Autodesk Inventor part; units mm, degrees
(part 2 of 2)
  line L250 (2.8637, 41.6829) -> (3.9176, 41.5971)
  arc A285 (2.2786, 42.8391) -> (2.0312, 43.0046) centre (2.0404, 42.7508) ccw
  line L251 (2.0312, 43.0046) -> (4.9529, 42.7667)
  arc A286 (4.9529, 42.7667) -> (4.682, 42.6434) centre (4.9028, 42.5177) ccw
  arc A287 (-0.6028, 41.7768) -> (-0.3767, 41.9297) centre (-0.6097, 42.0307) ccw
  arc A288 (-1.8939, 41.8886) -> (-1.6598, 41.7482) centre (-1.6667, 42.0021) ccw
  line L252 (-0.3767, 41.9297) -> (0.044, 42.8996)
  line L253 (-2.3665, 42.8343) -> (-1.8939, 41.8886)
  line L254 (-1.6598, 41.7482) -> (-0.6028, 41.7768)
  arc A289 (-2.3665, 42.8343) -> (-2.6303, 42.9721) centre (-2.5937, 42.7208) ccw
  line L255 (-2.6303, 42.9721) -> (0.3, 43.0515)
  arc A290 (0.3, 43.0515) -> (0.044, 42.8996) centre (0.277, 42.7985) ccw
  arc A291 (-5.1162, 41.4668) -> (-4.9079, 41.6431) centre (-5.1505, 41.7184) ccw
  arc A292 (-6.4117, 41.4383) -> (-6.1638, 41.324) centre (-6.1981, 41.5757) ccw
  line L256 (-4.9079, 41.6431) -> (-4.5945, 42.6529)
  line L257 (-6.9838, 42.3274) -> (-6.4117, 41.4383)
  line L258 (-6.1638, 41.324) -> (-5.1162, 41.4668)
  arc A293 (-6.9838, 42.3274) -> (-7.261, 42.4358) centre (-7.1974, 42.1899) ccw
  line L259 (-7.261, 42.4358) -> (-4.3565, 42.8316)
  arc A294 (-4.3565, 42.8316) -> (-4.5945, 42.6529) centre (-4.3519, 42.5776) ccw
  arc A295 (-9.5695, 40.6705) -> (-9.3815, 40.8684) centre (-9.6308, 40.917) ccw
  arc A296 (-10.8544, 40.5021) -> (-10.5956, 40.4153) centre (-10.6569, 40.6618) ccw
  line L260 (-9.3815, 40.8684) -> (-9.1792, 41.9061)
  line L261 (-11.5193, 41.3242) -> (-10.8544, 40.5021)
  line L262 (-10.5956, 40.4153) -> (-9.5695, 40.6705)
  arc A297 (-11.5193, 41.3242) -> (-11.8065, 41.402) centre (-11.7168, 41.1644) ccw
  line L263 (-11.8065, 41.402) -> (-8.9618, 42.1095)
  arc A298 (-8.9618, 42.1095) -> (-9.1792, 41.9061) centre (-8.9299, 41.8575) ccw
  arc A299 (-13.9107, 39.3975) -> (-13.7452, 39.6145) centre (-13.9983, 39.6359) ccw
  arc A300 (-15.1698, 39.0911) -> (-14.9032, 39.0328) centre (-14.9908, 39.2713) ccw
  line L264 (-13.7452, 39.6145) -> (-13.6562, 40.668)
  line L265 (-15.9197, 39.8365) -> (-15.1698, 39.0911)
  line L266 (-14.9032, 39.0328) -> (-13.9107, 39.3975)
  arc A301 (-15.9197, 39.8365) -> (-16.2137, 39.8828) centre (-16.0987, 39.6563) ccw
  line L267 (-16.2137, 39.8828) -> (-13.4621, 40.8937)
  arc A302 (-13.4621, 40.8937) -> (-13.6562, 40.668) centre (-13.4031, 40.6466) ccw
  arc A303 (-18.0888, 37.6625) -> (-17.9477, 37.8962) centre (-18.2016, 37.8901) ccw
  arc A304 (-19.3074, 37.2218) -> (-19.036, 37.1927) centre (-19.1489, 37.4203) ccw
  line L268 (-17.9477, 37.8962) -> (-17.9731, 38.9531)
  line L269 (-20.1334, 37.8817) -> (-19.3074, 37.2218)
  line L270 (-19.036, 37.1927) -> (-18.0888, 37.6625)
  arc A305 (-20.1334, 37.8817) -> (-20.4307, 37.896) centre (-20.292, 37.6833) ccw
  line L271 (-20.4307, 37.896) -> (-17.8046, 39.1985)
  arc A306 (-17.8046, 39.1985) -> (-17.9731, 38.9531) centre (-17.7192, 38.9592) ccw
  arc A307 (-22.0548, 35.486) -> (-21.9398, 35.7335) centre (-22.1916, 35.7) ccw
  arc A308 (-23.2186, 34.9161) -> (-22.9457, 34.9165) centre (-23.0825, 35.1305) ccw
  line L272 (-21.9398, 35.7335) -> (-22.0794, 36.7815)
  line L273 (-24.1111, 35.4828) -> (-23.2186, 34.9161)
  line L274 (-22.9457, 34.9165) -> (-22.0548, 35.486)
  arc A309 (-24.1111, 35.4828) -> (-24.4082, 35.4649) centre (-24.2473, 35.2684) ccw
  line L275 (-24.4082, 35.4649) -> (-21.9383, 37.0437)
  arc A310 (-21.9383, 37.0437) -> (-22.0794, 36.7815) centre (-21.8276, 36.8151) ccw
  arc A311 (-25.7622, 32.8934) -> (-25.6746, 33.152) centre (-25.9213, 33.0914) ccw
  arc A312 (-26.8576, 32.2011) -> (-26.5863, 32.231) centre (-26.7454, 32.429) ccw
  line L276 (-25.6746, 33.152) -> (-25.9267, 34.1787)
  line L277 (-27.8062, 32.668) -> (-26.8576, 32.2011)
  line L278 (-26.5863, 32.231) -> (-25.7622, 32.8934)
  arc A313 (-27.8062, 32.668) -> (-28.0996, 32.618) centre (-27.9183, 32.4401) ccw
  line L279 (-28.0996, 32.618) -> (-25.8149, 34.4545)
  arc A314 (-25.8149, 34.4545) -> (-25.9267, 34.1787) centre (-25.68, 34.2393) ccw
  point P0 (-30.4251, 30.4251)
  point P1 (-33.5363, 26.9572)
  point P2 (-36.2543, 23.1733)
  point P3 (-38.5472, 19.1177)
  point P4 (-40.3883, 14.8379)
  point P5 (-41.7558, 10.3842)
  point P6 (-42.6337, 5.8087)
  point P7 (-43.0118, 1.1652)
  point P8 (-42.8857, -3.4921)
  point P9 (-42.2567, -8.1084)
  point P10 (-41.1323, -12.6296)
  point P11 (-39.5257, -17.0027)
  point P12 (-37.4557, -21.1765)
  point P13 (-34.9465, -25.1021)
  point P14 (-32.0277, -28.7333)
  point P15 (-28.7333, -32.0277)
  point P16 (-25.1021, -34.9465)
  point P17 (-21.1765, -37.4557)
  point P18 (-17.0027, -39.5257)
  point P19 (-12.6296, -41.1323)
  point P20 (-8.1084, -42.2567)
  point P21 (-3.4921, -42.8857)
  point P22 (1.1652, -43.0118)
  point P23 (5.8087, -42.6337)
  point P24 (10.3842, -41.7558)
  point P25 (14.8379, -40.3883)
  point P26 (19.1177, -38.5472)
  point P27 (23.1733, -36.2543)
  point P28 (26.9572, -33.5363)
  point P29 (30.4251, -30.4251)
  point P30 (33.5363, -26.9572)
  point P31 (36.2543, -23.1733)
  point P32 (38.5472, -19.1177)
  point P33 (40.3883, -14.8379)
  point P34 (41.7558, -10.3842)
  point P35 (42.6337, -5.8087)
  point P36 (43.0118, -1.1652)
  point P37 (42.8857, 3.4921)
  point P38 (42.2567, 8.1084)
  point P39 (41.1323, 12.6296)
  point P40 (39.5257, 17.0027)
  point P41 (37.4557, 21.1765)
  point P42 (34.9465, 25.1021)
  point P43 (32.0277, 28.7333)
  point P44 (28.7333, 32.0277)
  point P45 (25.1021, 34.9465)
  point P46 (21.1765, 37.4557)
  point P47 (17.0027, 39.5257)
  point P48 (12.6296, 41.1323)
  point P49 (8.1084, 42.2567)
  point P50 (3.4921, 42.8857)
  point P51 (-1.1652, 43.0118)
  point P52 (-5.8087, 42.6337)
  point P53 (-10.3842, 41.7558)
  point P54 (-14.8379, 40.3883)
  point P55 (-19.1177, 38.5472)
  point P56 (-23.1733, 36.2543)
  point P57 (-26.9572, 33.5363)
  dimension "d40" = 0
  dimension "d41" = 0
  dimension "d42" = 0
  dimension "d43" = 0
  dimension "d44" = 0
  dimension "d45" = 0
  dimension "d47" = 43.0276
  dimension "d48" = 86.0552
  dimension "d49" = 0
  dimension "d50" = 0
  dimension "d51" = 0
  dimension "d54" = 360
  constraints: 624 point on circle, 560 end point, 314 centre point, 2 coincident, 1 concentric, 1 midpoint, 1219 other
  measures "d40" distance of point (0, 0) point (0, 0)
  measures "d41" distance of A0.centre point (0, 0)
  measures "d42" distance of point (0, 0) A0.centre
  measures "d43" distance of point (0, 0) A4.centre
  measures "d44" distance of point (0, 0) A4.centre
  measures "d45" distance of point (0, 0) point (0, 0)
  measures "d47" distance of A24.centre point (-30.425, 30.425)
  measures "d48" diameter of A81
  measures "d49" distance of A29.centre A24.centre
  measures "d50" distance of point (0, 0) A19.centre
  measures "d51" distance of point (0, 0) A24.centre
equation "\"d47\" = 0.5 * d48"
body "Solid1"
